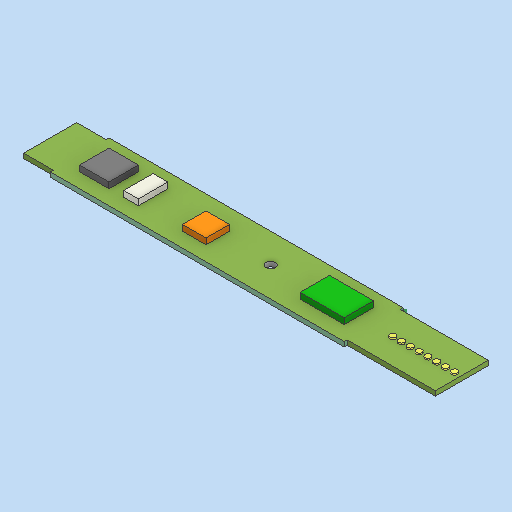
# Autodesk Inventor part: pcb板
Saved by Autodesk Inventor 2026.2 (Build 302298010, 298A)
## iProperties
Created: 2026-03-16
Part Number: pcb板
Material: 常规
Document SubType Name: Modeling
Designer: liu
Density: 1 g/cm^3
Appearance: 默认
Author: liu
Autodesk Inventor part; units mm, degrees
ref_plane "YZ Plane" through (0, 0, 0) normal (1, 0, 0) x (0, 1, 0)
ref_plane "XZ Plane" through (0, 0, 0) normal (0, 1, 0) x (-1, 0, 0)
ref_plane "XY Plane" through (0, 0, 0) normal (0, 0, 1) x (1, 0, 0)
sketch "草图1" plane through (0, 0, 0) normal (0, 1, 0) x (-1, 0, 0)
  line L0 (0, 20) -> (-100, 20)
  line L1 (-100, 20) -> (-100, 0)
  line L2 (-100, 0) -> (0, 0)
  line L3 (0, 0) -> (0, 20)
  point P0 (0, 0)
  dimension "d0" = 20
  dimension "d1" = 100
  constraints: 8 end point, 2 parallel, 1 coincident, 1 horizontal, 1 perpendicular
  measures "d0" distance of L2.end L0.start
  measures "d1" distance of L1.end L2.end
extrude "拉伸1" add sketch "草图1" along normal blind 1.6
sketch "草图2" plane through (0, 1.6, 0) normal (0, 1, 0) x (1, 0, 0)
  line L0 (5, -15) -> (15, -15)
  line L1 (15, -15) -> (15, -5)
  line L2 (15, -5) -> (5, -5)
  line L3 (5, -5) -> (5, -15)
  line L4 (100, 0) -> (0, 0) projected
  line L5 (0, 0) -> (0, -20) projected
  point P0 (0, 0)
  dimension "d4" = 10
  dimension "d5" = 10
  dimension "d6" = 5
  dimension "d7" = 5
  constraints: 8 end point, 2 parallel, 1 horizontal, 1 perpendicular
  measures "d4" distance of L2.end L0.start
  measures "d5" distance of L1.end L2.end
  measures "d6" distance between parallel lines of L2 L4
  measures "d7" distance between parallel lines of L3 L5
extrude "拉伸2" add sketch "草图2" along normal blind 2
sketch "草图3" plane through (0, 1.6, 0) normal (0, 1, 0) x (1, 0, 0)
  line L0 (80, -15) -> (95, -15)
  line L1 (95, -15) -> (95, -5)
  line L2 (95, -5) -> (80, -5)
  line L3 (80, -5) -> (80, -15)
  line L4 (100, 0) -> (0, 0) projected
  line L5 (100, -20) -> (100, 0) projected
  point P0 (0, 0)
  point P1 (100, -10)
  point P2 (95, -10)
  dimension "d10" = 10
  dimension "d11" = 15
  dimension "d12" = 5
  dimension "d13" = 5
  constraints: 8 end point, 2 midpoint, 2 parallel, 1 horizontal, 1 perpendicular
  measures "d10" distance of L2.end L0.start
  measures "d11" distance of L1.end L2.end
  measures "d12" distance between parallel lines of L2 L4
  measures "d13" distance of point (100, -10) point (95, -10)
extrude "拉伸3" add sketch "草图3" along normal blind 2
sketch "草图4" plane through (0, 1.6, 0) normal (0, 1, 0) x (1, 0, 0)
  line L0 (48, -15) -> (40, -15)
  line L1 (40, -15) -> (40, -7)
  line L2 (40, -7) -> (48, -7)
  line L3 (48, -7) -> (48, -15)
  line L4 (0, -20) -> (100, -20) projected
  line L5 (0, 0) -> (0, -20) projected
  point P0 (0, 0)
  point P1 (44, -15)
  dimension "d16" = 8
  dimension "d17" = 8
  dimension "d18" = 5
  dimension "d19" = 40
  constraints: 8 end point, 2 parallel, 1 horizontal, 1 midpoint, 1 perpendicular
  measures "d16" distance of L0.start L0.end
  measures "d17" distance of L0.end L1.end
  measures "d18" distance from line of L4 point (44, -15)
  measures "d19" distance between parallel lines of L5 L1
extrude "拉伸4" add sketch "草图4" along normal blind 2
sketch "草图5" plane through (0, 1.6, 0) normal (0, 1, 0) x (1, 0, 0)
  line L0 (25, -15) -> (20, -15)
  line L1 (20, -15) -> (20, -5)
  line L2 (20, -5) -> (25, -5)
  line L3 (25, -5) -> (25, -15)
  line L4 (0, -20) -> (100, -20) projected
  line L5 (0, 0) -> (0, -20) projected
  point P0 (0, 0)
  point P1 (20, -10)
  dimension "d22" = 5
  dimension "d23" = 10
  dimension "d24" = 5
  dimension "d25" = 20
  constraints: 8 end point, 2 parallel, 1 horizontal, 1 midpoint, 1 perpendicular
  measures "d22" distance of L0.start L0.end
  measures "d23" distance of L0.end L1.end
  measures "d24" distance between parallel lines of L4 L0
  measures "d25" distance from line of L5 point (20, -10)
extrude "拉伸5" add sketch "草图5" along normal blind 2
sketch "草图6" plane through (100, 0, 20) normal (1, 0, 0) x (0, 0, -1)
  point P0 (20, 0)
sketch "草图7" plane through (100, 0, 20) normal (1, 0, 0) x (0, 0, -1)
  line L0 (1, 0) -> (19, 0)
  line L1 (19, 0) -> (19, 1.6)
  line L2 (19, 1.6) -> (1, 1.6)
  line L3 (1, 1.6) -> (1, 0)
  line L4 (0, 0) -> (20, 0) projected
  line L5 (20, 0) -> (20, 1.6) projected
  point P0 (20, 0)
  point P1 (20, 0.8)
  dimension "d28" = 1.6
  dimension "d29" = 0
  dimension "d30" = 18
  dimension "d31" = 1
  constraints: 8 end point, 2 parallel, 1 horizontal, 1 midpoint, 1 perpendicular
  measures "d28" distance of L2.end L0.start
  measures "d29" distance between parallel lines of L4 L0
  measures "d30" distance of L1.end L2.end
  measures "d31" distance from line of point (20, 0.8) L1
extrude "拉伸6" add sketch "草图7" along normal blind 30
sketch "草图8" plane through (0, 0, 0) normal (-1, 0, 0) x (0, 0, 1)
  line L0 (1, 1.6) -> (19, 1.6)
  line L1 (19, 1.6) -> (19, 0)
  line L2 (19, 0) -> (1, 0)
  line L3 (1, 0) -> (1, 1.6)
  line L4 (0, 0) -> (20, 0) projected
  line L5 (20, 0) -> (20, 1.6) projected
  point P0 (0, 0)
  dimension "d34" = 1.6
  dimension "d35" = 0
  dimension "d36" = 18
  dimension "d37" = 1
  constraints: 8 end point, 2 parallel, 1 horizontal, 1 perpendicular
  measures "d34" distance of L0.end L1.end
  measures "d35" distance between parallel lines of L4 L2
  measures "d36" distance of L1.end L2.end
  measures "d37" distance between parallel lines of L5 L1
extrude "拉伸7" add sketch "草图8" along normal blind 10
sketch "草图9" plane through (0, 1.6, 0) normal (0, 1, 0) x (1, 0, 0)
  circle A0 centre (128, -10.5) radius 1
  line L0 (100, -1) -> (130, -1) projected
  line L1 (130, -1) -> (130, -19) projected
  circle A1 centre (125, -10.5) radius 1
  circle A2 centre (122, -10.5) radius 1
  circle A3 centre (119, -10.5) radius 1
  circle A4 centre (116, -10.5) radius 1
  circle A5 centre (113, -10.5) radius 1
  circle A6 centre (110, -10.5) radius 1
  circle A7 centre (107, -10.5) radius 1
  point P0 (0, 0)
  dimension "d40" = 2
  dimension "d41" = 9.5
  dimension "d42" = 2
  dimension "d45" = 3
  constraints: 8 centre point, 1 horizontal, 14 other
  measures "d40" diameter of A0
  measures "d41" distance from line of A0.centre L0
  measures "d42" distance from line of L1 A0.centre
  measures "d45" distance of A0.centre A1.centre
extrude "拉伸8" add sketch "草图9" along normal blind 0.5
sketch "草图10" plane through (0, 1.6, 0) normal (0, 1, 0) x (1, 0, 0)
  circle A0 centre (65, -10) radius 1.6
  line L0 (100, 0) -> (0, 0) projected
  line L1 (0, 0) -> (0, -1) projected
  point P0 (0, -0.5)
  dimension "d52" = 3.2
  dimension "d53" = 10
  dimension "d54" = 65
  constraints: 1 centre point, 1 midpoint
  measures "d52" diameter of A0
  measures "d53" distance from line of L0 A0.centre
  measures "d54" horizontal distance of point (0, -0.5) A0.centre
extrude "拉伸9" cut sketch "草图10" against normal blind 1.6
